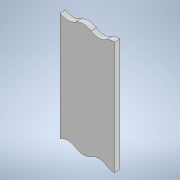
# Autodesk Inventor part: FlagPeiceVertical
Saved by Autodesk Inventor 2021 (Build 250183000, 183)
## iProperties
Created: 2021-03-22
Part Number: FlagPeiceVertical
Material: Générique
Document SubType Name: Modeling
Designer: turnb
Density: 1 g/cm^3
Appearance: Par défaut
Author: turnb
Autodesk Inventor part; units mm, degrees
ref_plane "YZ Plane" through (0, 0, 0) normal (1, 0, 0) x (0, 1, 0)
ref_plane "XZ Plane" through (0, 0, 0) normal (0, 1, 0) x (-1, 0, 0)
ref_plane "XY Plane" through (0, 0, 0) normal (0, 0, 1) x (1, 0, 0)
sketch "Esquisse1" plane through (0, 0, 0) normal (0, 0, 1) x (1, 0, 0)
  line L0 (150, -95.8007) -> (150, 95.8007)
  line L1 (-150, 100) -> (-150, -100)
  line L2 (-150, -100) -> (150, 100) construction
  line L3 (143.989, -95.9926) -> (-150, 100) construction
  line L4 (-50, 100) -> (-50, -100)
  line L5 (50, 100) -> (50, -100)
  arc A0 (-150, 100) -> (-121.6376, 100) centre (-135.8188, 121.2718) ccw
  line L6 (-150, 0) -> (150, 0)
  arc A1 (-121.6376, -100) -> (-150, -100) centre (-135.8188, -121.2718) ccw
  arc A2 (-93.2753, 100) -> (-121.6376, 100) centre (-107.4565, 78.7282) ccw
  arc A3 (-121.6376, -100) -> (-93.2753, -100) centre (-107.4565, -78.7282) ccw
  arc A4 (-93.2753, 100) -> (-64.9129, 100) centre (-79.0941, 121.2718) ccw
  arc A5 (-64.9129, -100) -> (-93.2753, -100) centre (-79.0941, -121.2718) ccw
  arc A6 (-36.5506, 100) -> (-64.9129, 100) centre (-50.7318, 78.7282) ccw
  arc A7 (-64.9129, -100) -> (-36.5506, -100) centre (-50.7318, -78.7282) ccw
  arc A8 (-36.5506, 100) -> (-8.1882, 100) centre (-22.3694, 121.2718) ccw
  arc A9 (-8.1882, -100) -> (-36.5506, -100) centre (-22.3694, -121.2718) ccw
  arc A10 (20.1741, 100) -> (-8.1882, 100) centre (5.9929, 78.7282) ccw
  arc A11 (-8.1882, -100) -> (20.1741, -100) centre (5.9929, -78.7282) ccw
  arc A12 (20.1741, 100) -> (48.5365, 100) centre (34.3553, 121.2718) ccw
  arc A13 (48.5365, -100) -> (20.1741, -100) centre (34.3553, -121.2718) ccw
  arc A14 (76.8988, 100) -> (48.5365, 100) centre (62.7176, 78.7282) ccw
  arc A15 (48.5365, -100) -> (76.8988, -100) centre (62.7176, -78.7282) ccw
  arc A16 (76.8988, 100) -> (105.2612, 100) centre (91.08, 121.2718) ccw
  arc A17 (105.2612, -100) -> (76.8988, -100) centre (91.08, -121.2718) ccw
  arc A18 (133.6235, 100) -> (105.2612, 100) centre (119.4423, 78.7282) ccw
  arc A19 (105.2612, -100) -> (133.6235, -100) centre (119.4423, -78.7282) ccw
  arc A20 (133.6235, 100) -> (150, 95.8007) centre (147.8047, 121.2718) ccw
  arc A21 (150, -95.8007) -> (133.6235, -100) centre (147.8047, -121.2718) ccw
  line L7 (-50, 100) -> (-50, 104.2832)
  line L8 (-50, -100) -> (-50, -104.2832)
  line L9 (50, -100) -> (50, -100.906)
  line L10 (50, 100) -> (50, 100.906)
  point P0 (0, 0)
  constraints: 49 point on circle, 22 centre point, 22 end point, 5 symmetric about line, 3 midpoint, 2 parallel, 2 vertical, 1 point on line, 1 tangent, 2 other
extrude "Extrusion1" add sketch "Esquisse1" along normal blind 10 contours L6 L1 A0 A2 A4 A6 L7 L4 | L4 L8 A7 A5 A3 A1 L1 L6
